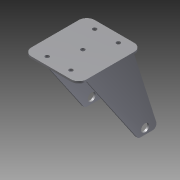
# Autodesk Inventor part: Rotation Caster Flange
Saved by Autodesk Inventor 2012 (Build 160160000, 160)
## iProperties
Created: 2011-10-20
Part Number: Rotation Caster Flange
Material: Aluminum-6061
Document SubType Name: Modeling
Designer: robotics
Density: 2.71 g/cm^3
Mass: 65.8499 g
Surface Area: 444.34 cm^2
Volume: 65.8499 cm^3
Author: robotics
Autodesk Inventor part; units mm, degrees
ref_plane "YZ Plane" through (0, 0, 0) normal (1, 0, 0) x (0, 1, 0)
ref_plane "XZ Plane" through (0, 0, 0) normal (0, 1, 0) x (-1, 0, 0)
ref_plane "XY Plane" through (0, 0, 0) normal (0, 0, 1) x (1, 0, 0)
sketch "Sketch2" plane through (0, 0, 0) normal (0, 1, 0) x (-1, 0, 0)
  line L0 (-44.45, 50.8) -> (44.45, 50.8)
  line L1 (44.45, 50.8) -> (44.45, -50.8)
  line L2 (44.45, -50.8) -> (-44.45, -50.8)
  line L3 (-44.45, -50.8) -> (-44.45, 50.8)
  point P0 (0, 0)
  dimension "d0" = 44.45
  dimension "d1" = 44.45
  dimension "d2" = 50.8
  dimension "d3" = 50.8
  constraints: 8 end point, 2 parallel, 1 horizontal, 1 perpendicular
  measures "d0" distance from line of L1 point (0, 0)
  measures "d1" distance from line of L3 point (0, 0)
  measures "d2" distance from line of L0 point (0, 0)
  measures "d3" distance from line of L2 point (0, 0)
extrude "Extrusion1" add sketch "Sketch2" along normal blind 3.175
fillet "Fillet1" radius 12.7 4 edges at (44.45, 1.5875, 50.8) (-44.45, 1.5875, 50.8) (44.45, 1.5875, -50.8) (-44.45, 1.5875, -50.8)
sketch "Sketch3" plane through (0, 3.175, 0) normal (0, 1, 0) x (1, 0, 0)
  line L0 (-19.05, 38.1) -> (19.05, 38.1) construction
  line L1 (19.05, 38.1) -> (19.05, -38.1) construction
  line L2 (19.05, -38.1) -> (-19.05, -38.1) construction
  line L3 (-19.05, -38.1) -> (-19.05, 38.1) construction
  point P0 (0, 0)
  point P1 (0, 0)
  point P2 (-19.05, 0)
  point P3 (0, 38.1)
  dimension "d36" = 38.1
  dimension "d37" = 76.2
  constraints: 8 end point, 3 horizontal alignment, 3 vertical alignment, 2 midpoint, 2 parallel, 1 coincident, 1 horizontal, 1 perpendicular
  measures "d36" distance of L0.start L0.end
  measures "d37" distance of L2.end L0.start
hole "Hole1" at (-19.05, 3.175, -38.1) at (19.05, 3.175, -38.1) at (19.05, 3.175, 38.1) at (-19.05, 3.175, 38.1) at (0, 3.175, 0) direction (0, -1, 0) diameter 6.35 end through all
sketch "Sketch4" plane through (0, 0, 0) normal (0, -1, 0) x (1, 0, 0)
  circle A0 centre (-19.05, 38.1) radius 3.175 projected
  line L0 (44.45, -38.1) -> (44.45, 38.1) projected
  line L1 (-44.45, 38.1) -> (-44.45, -38.1) projected
  line L2 (44.45, 38.1) -> (41.275, 38.1)
  line L3 (41.275, 38.1) -> (41.275, -88.9)
  line L4 (41.275, -88.9) -> (44.45, -88.9)
  line L5 (44.45, -88.9) -> (44.45, 38.1)
  line L6 (-44.45, 38.1) -> (-41.275, 38.1)
  line L7 (-41.275, 38.1) -> (-41.275, -88.9)
  line L8 (-41.275, -88.9) -> (-44.45, -88.9)
  line L9 (-44.45, -88.9) -> (-44.45, 38.1)
  dimension "d18" = 3.175
  dimension "d19" = 3.175
  dimension "d20" = 127
  dimension "d21" = 127
  constraints: 16 end point, 4 parallel, 2 horizontal, 2 horizontal alignment, 2 perpendicular, 2 point on line
  measures "d18" distance of L6.start L6.end
  measures "d19" distance of L2.start L2.end
  measures "d20" distance of L2.end L3.end
  measures "d21" distance of L6.end L7.end
extrude "Extrusion2" add sketch "Sketch4" along normal blind 120.65 contours L5 L4 L3 L2 L0 | L6 L7 L8 L9 L1
sketch "Sketch5" plane through (44.45, 3.175, 38.1) normal (1, 0, 0) x (0, 0, -1)
  line L0 (0, -3.175) -> (0, -123.825) projected
  line L1 (0, -3.175) -> (82.55, -123.825)
  line L2 (76.2, -3.175) -> (114.3, -123.825)
  line L3 (0, -3.175) -> (0, -123.825)
  line L4 (82.55, -123.825) -> (0, -123.825)
  line L5 (0, -123.825) -> (127, -123.825) projected
  line L6 (127, -3.175) -> (76.2, -3.175) projected
  line L7 (76.2, 0) -> (76.2, -3.175) projected
  line L8 (127, -3.175) -> (127, -123.825) projected
  point P0 (38.1, -3.175)
  dimension "d39" = 31.75
  dimension "d40" = 12.7
  constraints: 8 end point, 2 point on line, 1 collinear, 1 perpendicular
  measures "d39" distance of L2.end L1.end
  measures "d40" distance of L5.end L2.end
extrude "Extrusion3" cut sketch "Sketch5" against normal blind 127
sketch "Sketch6" plane through (44.45, 3.175, 38.1) normal (1, 0, 0) x (0, 0, -1)
  line L0 (82.55, -123.825) -> (114.3, -123.825) projected
  line L1 (98.425, -123.825) -> (38.1, -3.175) construction
  point P0 (93.6625, -114.3)
  dimension "d41" = 9.525
  constraints: 2 end point, 1 midpoint, 1 point on line
  measures "d41" distance from line of L0 point (93.662, -114.3)
hole "Hole2" at (44.45, -111.125, -55.5625) direction (-1, 0, 0) diameter 12.7 end through all
fillet "Fillet2" radius 6.35 4 edges at (42.8625, -120.65, -44.45) (-42.8625, -120.65, -44.45) (-42.8625, -120.65, -76.2) (42.8625, -120.65, -76.2)
equation "\"d1\" = d0"
equation "\"d3\" = d2"
equation "\"d4\" = metalThickness"
equation "\"d18\" = metalThickness"
equation "\"d19\" = metalThickness"
equation "\"d21\" = d20"
equation "\"metalThickness\" = 3.175"
body "Solid1"
